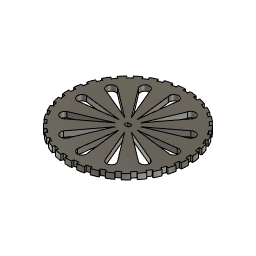
Drive wheel 1 v1 (Autodesk Fusion 360 design; units mm, degrees)
Autodesk Fusion 360 part; units mm, degrees
sketch "Sketch1" plane through (0, 0, 0) normal (0, 0, 1) x (1, 0, 0)
  circle A0 centre (0, 0) radius 65
  dimension "d1" = 130
  constraint coincident A0.centre origin
  measures "d1" diameter of A0
extrude "Extrude1" add sketch "Sketch1" along normal blind 6
sketch "Sketch2" plane through (0, 0, 6) normal (0, 0, 1) x (-1, 0, 0)
  circle A0 centre (0, 0) radius 65
  line L0 (2.5, -62.5) -> (-2.5, -62.5)
  line L1 (-2.5, -62.5) -> (-2.5, -64.9519)
  line L2 (2.5, -64.9519) -> (2.5, -62.5)
  line L3 (2.5, -62.5) -> (0, -65) construction
  line L4 (-2.5, -62.5) -> (0, -65) construction
  line L5 (2.5, -65) -> (2.5, -62.5)
  constraint horizontal L0
  constraint perpendicular L0 L1
  constraint parallel L1 L2
  constraint coincident A0 L3.end
  constraint coincident A0 L2.start
  constraint coincident L2 L5.start
  constraint coincident A0 L1.end
extrude "Extrude2" cut sketch "Sketch2" against normal blind 6 contours A0 L0 L1 L2 L5 picked at (0.2778, -63.3316)
pattern_circular "C-Pattern1" count 33 over 360 about axis through (0, 0, 1.75) along (0, 0, 1) of "Extrude2"
sketch "Sketch3" plane through (0, 0, 6) normal (0, 0, 1) x (-1, 0, 0)
  line L0 (-9.3734, -61.8437) -> (-9.8374, -64.2513)
  arc A0 (-9.8374, -64.2513) -> (-2.5, -64.9519) centre (0, 0) ccw
  line L1 (-2.5, -64.9519) -> (-2.5, -62.5)
  line L2 (-2.5, -62.5) -> (2.5, -62.5)
  line L3 (2.5, -62.5) -> (2.5, -64.9519)
  arc A1 (2.5, -64.9519) -> (9.8374, -64.2513) centre (0, 0) ccw
  line L4 (9.8374, -64.2513) -> (9.3734, -61.8437)
  line L5 (9.3734, -61.8437) -> (14.283, -60.8974)
  line L6 (14.283, -60.8974) -> (14.7471, -63.305)
  arc A2 (14.7471, -63.305) -> (21.8193, -61.2284) centre (0, 0) ccw
  line L7 (21.8193, -61.2284) -> (20.908, -58.9522)
  line L8 (20.908, -58.9522) -> (25.5498, -57.0938)
  line L9 (25.5498, -57.0938) -> (26.4611, -59.3701)
  arc A3 (26.4611, -59.3701) -> (33.0125, -55.9926) centre (0, 0) ccw
  line L10 (33.0125, -55.9926) -> (31.6869, -53.9299)
  line L11 (31.6869, -53.9299) -> (35.8932, -51.2267)
  line L12 (35.8932, -51.2267) -> (37.2188, -53.2894)
  arc A4 (37.2188, -53.2894) -> (43.0126, -48.7331) centre (0, 0) ccw
  line L13 (43.0126, -48.7331) -> (41.3206, -46.9586)
  line L14 (41.3206, -46.9586) -> (44.9393, -43.5082)
  line L15 (44.9393, -43.5082) -> (46.6313, -45.2827)
  arc A5 (46.6313, -45.2827) -> (51.4581, -39.7122) centre (0, 0) ccw
  line L16 (51.4581, -39.7122) -> (49.4609, -38.29)
  line L17 (49.4609, -38.29) -> (52.3611, -34.2171)
  line L18 (52.3611, -34.2171) -> (54.3584, -35.6394)
  arc A6 (54.3584, -35.6394) -> (58.0438, -29.2561) centre (0, 0) ccw
  line L19 (58.0438, -29.2561) -> (55.8135, -28.2375)
  line L20 (55.8135, -28.2375) -> (57.8905, -23.6894)
  line L21 (57.8905, -23.6894) -> (60.1209, -24.7079)
  arc A7 (60.1209, -24.7079) -> (62.5316, -17.7425) centre (0, 0) ccw
  line L22 (62.5316, -17.7425) -> (60.1488, -17.1645)
  line L23 (60.1488, -17.1645) -> (61.3276, -12.3054)
  line L24 (61.3276, -12.3054) -> (63.7104, -12.8835)
  arc A8 (63.7104, -12.8835) -> (64.7594, -5.5877) centre (0, 0) ccw
  line L25 (64.7594, -5.5877) -> (62.3103, -5.471)
  line L26 (62.3103, -5.471) -> (62.5482, -0.4767)
  line L27 (62.5482, -0.4767) -> (64.9973, -0.5934)
  arc A9 (64.9973, -0.5934) -> (64.6466, 6.7691) centre (0, 0) ccw
  line L28 (64.6466, 6.7691) -> (62.2196, 6.4201)
  line L29 (62.2196, 6.4201) -> (61.5081, 11.3692)
  line L30 (61.5081, 11.3692) -> (63.935, 11.7182)
  arc A10 (63.935, 11.7182) -> (62.1973, 18.8812) centre (0, 0) ccw
  line L31 (62.1973, 18.8812) -> (59.8802, 18.0792)
  line L32 (59.8802, 18.0792) -> (58.2449, 22.8043)
  line L33 (58.2449, 22.8043) -> (60.5619, 23.6062)
  arc A11 (60.5619, 23.6062) -> (57.5, 30.3109) centre (0, 0) ccw
  line L34 (57.5, 30.3109) -> (55.3766, 29.0849)
  line L35 (55.3766, 29.0849) -> (52.8766, 33.4151)
  line L36 (52.8766, 33.4151) -> (55, 34.641)
  arc A12 (55, 34.641) -> (50.7245, 40.6451) centre (0, 0) ccw
  line L37 (50.7245, 40.6451) -> (48.8715, 39.0394)
  line L38 (48.8715, 39.0394) -> (45.5972, 42.8182)
  line L39 (45.5972, 42.8182) -> (47.4502, 44.4238)
  arc A13 (47.4502, 44.4238) -> (42.1157, 49.5102) centre (0, 0) ccw
  line L40 (42.1157, 49.5102) -> (40.6001, 47.5829)
  line L41 (40.6001, 47.5829) -> (36.6698, 50.6737)
  line L42 (36.6698, 50.6737) -> (38.1855, 52.601)
  arc A14 (38.1855, 52.601) -> (31.9848, 56.586) centre (0, 0) ccw
  line L43 (31.9848, 56.586) -> (30.8612, 54.4067)
  line L44 (30.8612, 54.4067) -> (26.4171, 56.6978)
  line L45 (26.4171, 56.6978) -> (27.5406, 58.8771)
  arc A15 (27.5406, 58.8771) -> (20.6978, 61.6166) centre (0, 0) ccw
  line L46 (20.6978, 61.6166) -> (20.007, 59.264)
  line L47 (20.007, 59.264) -> (15.2096, 60.6726)
  line L48 (15.2096, 60.6726) -> (15.9003, 63.0252)
  arc A16 (15.9003, 63.0252) -> (8.6628, 64.4202) centre (0, 0) ccw
  line L49 (8.6628, 64.4202) -> (8.4297, 61.9794)
  line L50 (8.4297, 61.9794) -> (3.4523, 62.4546)
  line L51 (3.4523, 62.4546) -> (3.6854, 64.8954)
  arc A17 (3.6854, 64.8954) -> (-3.6854, 64.8954) centre (0, 0) ccw
  line L52 (-3.6854, 64.8954) -> (-3.4523, 62.4546)
  line L53 (-3.4523, 62.4546) -> (-8.4297, 61.9794)
  line L54 (-8.4297, 61.9794) -> (-8.6628, 64.4202)
  arc A18 (-8.6628, 64.4202) -> (-15.9003, 63.0252) centre (0, 0) ccw
  line L55 (-15.9003, 63.0252) -> (-15.2096, 60.6726)
  line L56 (-15.2096, 60.6726) -> (-20.007, 59.264)
  line L57 (-20.007, 59.264) -> (-20.6978, 61.6166)
  arc A19 (-20.6978, 61.6166) -> (-27.5406, 58.8771) centre (0, 0) ccw
  line L58 (-27.5406, 58.8771) -> (-26.4171, 56.6978)
  line L59 (-26.4171, 56.6978) -> (-30.8612, 54.4067)
  line L60 (-30.8612, 54.4067) -> (-31.9848, 56.586)
  arc A20 (-31.9848, 56.586) -> (-38.1855, 52.601) centre (0, 0) ccw
  line L61 (-38.1855, 52.601) -> (-36.6698, 50.6737)
  line L62 (-36.6698, 50.6737) -> (-40.6001, 47.5829)
  line L63 (-40.6001, 47.5829) -> (-42.1157, 49.5102)
  arc A21 (-42.1157, 49.5102) -> (-47.4502, 44.4238) centre (0, 0) ccw
  line L64 (-47.4502, 44.4238) -> (-45.5972, 42.8182)
  line L65 (-45.5972, 42.8182) -> (-48.8715, 39.0394)
  line L66 (-48.8715, 39.0394) -> (-50.7245, 40.6451)
  arc A22 (-50.7245, 40.6451) -> (-55, 34.641) centre (0, 0) ccw
  line L67 (-55, 34.641) -> (-52.8766, 33.4151)
  line L68 (-52.8766, 33.4151) -> (-55.3766, 29.0849)
  line L69 (-55.3766, 29.0849) -> (-57.5, 30.3109)
  arc A23 (-57.5, 30.3109) -> (-60.5619, 23.6062) centre (0, 0) ccw
  line L70 (-60.5619, 23.6062) -> (-58.2449, 22.8043)
  line L71 (-58.2449, 22.8043) -> (-59.8802, 18.0792)
  line L72 (-59.8802, 18.0792) -> (-62.1973, 18.8812)
  arc A24 (-62.1973, 18.8812) -> (-63.935, 11.7182) centre (0, 0) ccw
  line L73 (-63.935, 11.7182) -> (-61.5081, 11.3692)
  line L74 (-61.5081, 11.3692) -> (-62.2196, 6.4201)
  line L75 (-62.2196, 6.4201) -> (-64.6466, 6.7691)
  arc A25 (-64.6466, 6.7691) -> (-64.9973, -0.5934) centre (0, 0) ccw
  line L76 (-64.9973, -0.5934) -> (-62.5482, -0.4767)
  line L77 (-62.5482, -0.4767) -> (-62.3103, -5.471)
  line L78 (-62.3103, -5.471) -> (-64.7594, -5.5877)
  arc A26 (-64.7594, -5.5877) -> (-63.7104, -12.8835) centre (0, 0) ccw
  line L79 (-63.7104, -12.8835) -> (-61.3276, -12.3054)
  line L80 (-61.3276, -12.3054) -> (-60.1488, -17.1645)
  line L81 (-60.1488, -17.1645) -> (-62.5316, -17.7425)
  arc A27 (-62.5316, -17.7425) -> (-60.1209, -24.7079) centre (0, 0) ccw
  line L82 (-60.1209, -24.7079) -> (-57.8905, -23.6894)
  line L83 (-57.8905, -23.6894) -> (-55.8135, -28.2375)
  line L84 (-55.8135, -28.2375) -> (-58.0438, -29.2561)
  arc A28 (-58.0438, -29.2561) -> (-54.3584, -35.6394) centre (0, 0) ccw
  line L85 (-54.3584, -35.6394) -> (-52.3611, -34.2171)
  line L86 (-52.3611, -34.2171) -> (-49.4609, -38.29)
  line L87 (-49.4609, -38.29) -> (-51.4581, -39.7122)
  arc A29 (-51.4581, -39.7122) -> (-46.6313, -45.2827) centre (0, 0) ccw
  line L88 (-46.6313, -45.2827) -> (-44.9393, -43.5082)
  line L89 (-44.9393, -43.5082) -> (-41.3206, -46.9586)
  line L90 (-41.3206, -46.9586) -> (-43.0126, -48.7331)
  arc A30 (-43.0126, -48.7331) -> (-37.2188, -53.2894) centre (0, 0) ccw
  line L91 (-37.2188, -53.2894) -> (-35.8932, -51.2267)
  line L92 (-35.8932, -51.2267) -> (-31.6869, -53.9299)
  line L93 (-31.6869, -53.9299) -> (-33.0125, -55.9926)
  arc A31 (-33.0125, -55.9926) -> (-26.4611, -59.3701) centre (0, 0) ccw
  line L94 (-26.4611, -59.3701) -> (-25.5498, -57.0938)
  line L95 (-25.5498, -57.0938) -> (-20.908, -58.9522)
  line L96 (-20.908, -58.9522) -> (-21.8193, -61.2284)
  arc A32 (-21.8193, -61.2284) -> (-14.7471, -63.305) centre (0, 0) ccw
  line L97 (-14.7471, -63.305) -> (-14.283, -60.8974)
  line L98 (-14.283, -60.8974) -> (-9.3734, -61.8437)
  circle A33 centre (0, 0) radius 2.75
  line L99 (25, -1.85) -> (-25, -1.85)
  line L100 (-25, -1.85) -> (-25, 1.85)
  line L101 (-25, 1.85) -> (25, 1.85)
  line L102 (25, 1.85) -> (25, -1.85)
  line L103 (25, -1.85) -> (-25, 1.85) construction
  line L104 (-25, -1.85) -> (25, 1.85) construction
  dimension "d12" = 5.5
  dimension "d13" = 3.7
  constraint concentric A0 A33
  constraint horizontal L99
  constraint perpendicular L99 L100
  constraint parallel L99 L101
  constraint parallel L100 L102
  constraint coincident L103 A0.centre
  constraint coincident L104 A0.centre
  constraint coincident A0.centre A1.centre
  measures "d12" diameter of A33
  measures "d13" distance of L99.end L100.end
extrude "Extrude4" cut sketch "Sketch3" against normal blind 6 contours A33 L99 L101
sketch "Sketch4" plane through (0, 0, 0) normal (0, 0, -1) x (1, 0, 0)
  line L0 (-2.0347, 1.85) -> (2.0347, 1.85)
  arc A0 (2.0347, -1.85) -> (2.0347, 1.85) centre (0, 0) ccw
  line L1 (2.0347, -1.85) -> (-2.0347, -1.85)
  arc A1 (-2.0347, 1.85) -> (-2.0347, -1.85) centre (0, 0) ccw
  line L2 (9.8374, -64.2513) -> (9.3734, -61.8437)
  line L3 (9.3734, -61.8437) -> (14.283, -60.8974)
  line L4 (14.283, -60.8974) -> (14.7471, -63.305)
  arc A2 (14.7471, -63.305) -> (21.8193, -61.2284) centre (0, 0) ccw
  line L5 (21.8193, -61.2284) -> (20.908, -58.9522)
  line L6 (20.908, -58.9522) -> (25.5498, -57.0938)
  line L7 (25.5498, -57.0938) -> (26.4611, -59.3701)
  arc A3 (26.4611, -59.3701) -> (33.0125, -55.9926) centre (0, 0) ccw
  line L8 (33.0125, -55.9926) -> (31.6869, -53.9299)
  line L9 (31.6869, -53.9299) -> (35.8932, -51.2267)
  line L10 (35.8932, -51.2267) -> (37.2188, -53.2894)
  arc A4 (37.2188, -53.2894) -> (43.0126, -48.7331) centre (0, 0) ccw
  line L11 (43.0126, -48.7331) -> (41.3206, -46.9586)
  line L12 (41.3206, -46.9586) -> (44.9393, -43.5082)
  line L13 (44.9393, -43.5082) -> (46.6313, -45.2827)
  arc A5 (46.6313, -45.2827) -> (51.4581, -39.7122) centre (0, 0) ccw
  line L14 (51.4581, -39.7122) -> (49.4609, -38.29)
  line L15 (49.4609, -38.29) -> (52.3611, -34.2171)
  line L16 (52.3611, -34.2171) -> (54.3584, -35.6394)
  arc A6 (54.3584, -35.6394) -> (58.0438, -29.2561) centre (0, 0) ccw
  line L17 (58.0438, -29.2561) -> (55.8135, -28.2375)
  line L18 (55.8135, -28.2375) -> (57.8905, -23.6894)
  line L19 (57.8905, -23.6894) -> (60.1209, -24.7079)
  arc A7 (60.1209, -24.7079) -> (62.5316, -17.7425) centre (0, 0) ccw
  line L20 (62.5316, -17.7425) -> (60.1488, -17.1645)
  line L21 (60.1488, -17.1645) -> (61.3276, -12.3054)
  line L22 (61.3276, -12.3054) -> (63.7104, -12.8835)
  arc A8 (63.7104, -12.8835) -> (64.7594, -5.5877) centre (0, 0) ccw
  line L23 (64.7594, -5.5877) -> (62.3103, -5.471)
  line L24 (62.3103, -5.471) -> (62.5482, -0.4767)
  line L25 (62.5482, -0.4767) -> (64.9973, -0.5934)
  arc A9 (64.9973, -0.5934) -> (64.6466, 6.7691) centre (0, 0) ccw
  line L26 (64.6466, 6.7691) -> (62.2196, 6.4201)
  line L27 (62.2196, 6.4201) -> (61.5081, 11.3692)
  line L28 (61.5081, 11.3692) -> (63.935, 11.7182)
  arc A10 (63.935, 11.7182) -> (62.1973, 18.8812) centre (0, 0) ccw
  line L29 (62.1973, 18.8812) -> (59.8802, 18.0792)
  line L30 (59.8802, 18.0792) -> (58.2449, 22.8043)
  line L31 (58.2449, 22.8043) -> (60.5619, 23.6062)
  arc A11 (60.5619, 23.6062) -> (57.5, 30.3109) centre (0, 0) ccw
  line L32 (57.5, 30.3109) -> (55.3766, 29.0849)
  line L33 (55.3766, 29.0849) -> (52.8766, 33.4151)
  line L34 (52.8766, 33.4151) -> (55, 34.641)
  arc A12 (55, 34.641) -> (50.7245, 40.6451) centre (0, 0) ccw
  line L35 (50.7245, 40.6451) -> (48.8715, 39.0394)
  line L36 (48.8715, 39.0394) -> (45.5972, 42.8182)
  line L37 (45.5972, 42.8182) -> (47.4502, 44.4238)
  arc A13 (47.4502, 44.4238) -> (42.1157, 49.5102) centre (0, 0) ccw
  line L38 (42.1157, 49.5102) -> (40.6001, 47.5829)
  line L39 (40.6001, 47.5829) -> (36.6698, 50.6737)
  line L40 (36.6698, 50.6737) -> (38.1855, 52.601)
  arc A14 (38.1855, 52.601) -> (31.9848, 56.586) centre (0, 0) ccw
  line L41 (31.9848, 56.586) -> (30.8612, 54.4067)
  line L42 (30.8612, 54.4067) -> (26.4171, 56.6978)
  line L43 (26.4171, 56.6978) -> (27.5406, 58.8771)
  arc A15 (27.5406, 58.8771) -> (20.6978, 61.6166) centre (0, 0) ccw
  line L44 (20.6978, 61.6166) -> (20.007, 59.264)
  line L45 (20.007, 59.264) -> (15.2096, 60.6726)
  line L46 (15.2096, 60.6726) -> (15.9003, 63.0252)
  arc A16 (15.9003, 63.0252) -> (8.6628, 64.4202) centre (0, 0) ccw
  line L47 (8.6628, 64.4202) -> (8.4297, 61.9794)
  line L48 (8.4297, 61.9794) -> (3.4523, 62.4546)
  line L49 (3.4523, 62.4546) -> (3.6854, 64.8954)
  arc A17 (3.6854, 64.8954) -> (-3.6854, 64.8954) centre (0, 0) ccw
  line L50 (-3.6854, 64.8954) -> (-3.4523, 62.4546)
  line L51 (-3.4523, 62.4546) -> (-8.4297, 61.9794)
  line L52 (-8.4297, 61.9794) -> (-8.6628, 64.4202)
  arc A18 (-8.6628, 64.4202) -> (-15.9003, 63.0252) centre (0, 0) ccw
  line L53 (-15.9003, 63.0252) -> (-15.2096, 60.6726)
  line L54 (-15.2096, 60.6726) -> (-20.007, 59.264)
  line L55 (-20.007, 59.264) -> (-20.6978, 61.6166)
  arc A19 (-20.6978, 61.6166) -> (-27.5406, 58.8771) centre (0, 0) ccw
  line L56 (-27.5406, 58.8771) -> (-26.4171, 56.6978)
  line L57 (-26.4171, 56.6978) -> (-30.8612, 54.4067)
  line L58 (-30.8612, 54.4067) -> (-31.9848, 56.586)
  arc A20 (-31.9848, 56.586) -> (-38.1855, 52.601) centre (0, 0) ccw
  line L59 (-38.1855, 52.601) -> (-36.6698, 50.6737)
  line L60 (-36.6698, 50.6737) -> (-40.6001, 47.5829)
  line L61 (-40.6001, 47.5829) -> (-42.1157, 49.5102)
  arc A21 (-42.1157, 49.5102) -> (-47.4502, 44.4238) centre (0, 0) ccw
  line L62 (-47.4502, 44.4238) -> (-45.5972, 42.8182)
  line L63 (-45.5972, 42.8182) -> (-48.8715, 39.0394)
  line L64 (-48.8715, 39.0394) -> (-50.7245, 40.6451)
  arc A22 (-50.7245, 40.6451) -> (-55, 34.641) centre (0, 0) ccw
  line L65 (-55, 34.641) -> (-52.8766, 33.4151)
  line L66 (-52.8766, 33.4151) -> (-55.3766, 29.0849)
  line L67 (-55.3766, 29.0849) -> (-57.5, 30.3109)
  arc A23 (-57.5, 30.3109) -> (-60.5619, 23.6062) centre (0, 0) ccw
  line L68 (-60.5619, 23.6062) -> (-58.2449, 22.8043)
  line L69 (-58.2449, 22.8043) -> (-59.8802, 18.0792)
  line L70 (-59.8802, 18.0792) -> (-62.1973, 18.8812)
  arc A24 (-62.1973, 18.8812) -> (-63.935, 11.7182) centre (0, 0) ccw
  line L71 (-63.935, 11.7182) -> (-61.5081, 11.3692)
  line L72 (-61.5081, 11.3692) -> (-62.2196, 6.4201)
  line L73 (-62.2196, 6.4201) -> (-64.6466, 6.7691)
  arc A25 (-64.6466, 6.7691) -> (-64.9973, -0.5934) centre (0, 0) ccw
  line L74 (-64.9973, -0.5934) -> (-62.5482, -0.4767)
  line L75 (-62.5482, -0.4767) -> (-62.3103, -5.471)
  line L76 (-62.3103, -5.471) -> (-64.7594, -5.5877)
  arc A26 (-64.7594, -5.5877) -> (-63.7104, -12.8835) centre (0, 0) ccw
  line L77 (-63.7104, -12.8835) -> (-61.3276, -12.3054)
  line L78 (-61.3276, -12.3054) -> (-60.1488, -17.1645)
  line L79 (-60.1488, -17.1645) -> (-62.5316, -17.7425)
  arc A27 (-62.5316, -17.7425) -> (-60.1209, -24.7079) centre (0, 0) ccw
  line L80 (-60.1209, -24.7079) -> (-57.8905, -23.6894)
  line L81 (-57.8905, -23.6894) -> (-55.8135, -28.2375)
  line L82 (-55.8135, -28.2375) -> (-58.0438, -29.2561)
  arc A28 (-58.0438, -29.2561) -> (-54.3584, -35.6394) centre (0, 0) ccw
  line L83 (-54.3584, -35.6394) -> (-52.3611, -34.2171)
  line L84 (-52.3611, -34.2171) -> (-49.4609, -38.29)
  line L85 (-49.4609, -38.29) -> (-51.4581, -39.7122)
  arc A29 (-51.4581, -39.7122) -> (-46.6313, -45.2827) centre (0, 0) ccw
  line L86 (-46.6313, -45.2827) -> (-44.9393, -43.5082)
  line L87 (-44.9393, -43.5082) -> (-41.3206, -46.9586)
  line L88 (-41.3206, -46.9586) -> (-43.0126, -48.7331)
  arc A30 (-43.0126, -48.7331) -> (-37.2188, -53.2894) centre (0, 0) ccw
  line L89 (-37.2188, -53.2894) -> (-35.8932, -51.2267)
  line L90 (-35.8932, -51.2267) -> (-31.6869, -53.9299)
  line L91 (-31.6869, -53.9299) -> (-33.0125, -55.9926)
  arc A31 (-33.0125, -55.9926) -> (-26.4611, -59.3701) centre (0, 0) ccw
  line L92 (-26.4611, -59.3701) -> (-25.5498, -57.0938)
  line L93 (-25.5498, -57.0938) -> (-20.908, -58.9522)
  line L94 (-20.908, -58.9522) -> (-21.8193, -61.2284)
  arc A32 (-21.8193, -61.2284) -> (-14.7471, -63.305) centre (0, 0) ccw
  line L95 (-14.7471, -63.305) -> (-14.283, -60.8974)
  line L96 (-14.283, -60.8974) -> (-9.3734, -61.8437)
  line L97 (-9.3734, -61.8437) -> (-9.8374, -64.2513)
  arc A33 (-9.8374, -64.2513) -> (-2.5, -64.9519) centre (0, 0) ccw
  line L98 (-2.5, -64.9519) -> (-2.5, -62.5)
  line L99 (-2.5, -62.5) -> (2.5, -62.5)
  line L100 (2.5, -62.5) -> (2.5, -64.9519)
  arc A34 (2.5, -64.9519) -> (9.8374, -64.2513) centre (0, 0) ccw
  circle A35 centre (0, 50) radius 5
  line L101 (-5, 50) -> (-0.0386, 10.3089)
  line L102 (-0.0386, 10.3089) -> (4.9988, 49.9904)
  dimension "d16" = 10
  dimension "d17" = 40
  dimension "d18" = 40
  constraint coincident A35 L101.start
  measures "d16" diameter of A35
  measures "d17" distance of L101.start L101.end
  measures "d18" distance of L101.end L102.end
extrude "Extrude5" cut sketch "Sketch4" against normal blind 6 contours A35 L101 L102 | A35 L102 | A35 L101 L102
pattern_circular "C-Pattern2" count 12 over 360 about axis through (0, 0, 1.75) along (0, 0, 1) of "Extrude5"
